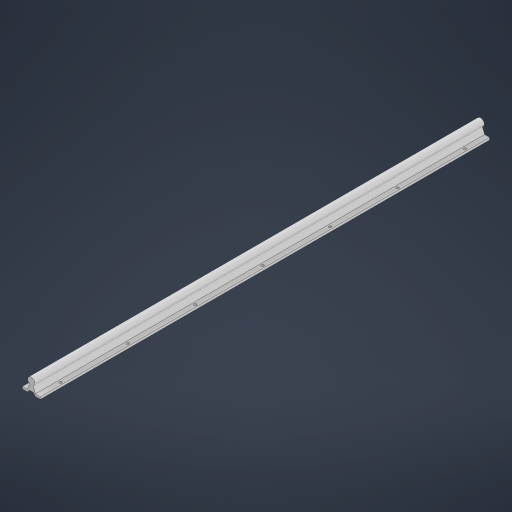
# Autodesk Inventor part: Linear Rail
Saved by Autodesk Inventor 2024 (Build 280153000, 153)
## iProperties
Created: 2024-10-26
Part Number: Linear Rail
Material: Generic
Document SubType Name: Modeling
Designer: jerem
Density: 1 g/cm^3
Appearance: Default
Author: jerem
Autodesk Inventor part; units mm, degrees
ref_plane "YZ Plane" through (0, 0, 0) normal (1, 0, 0) x (0, 1, 0)
ref_plane "XZ Plane" through (0, 0, 0) normal (0, 1, 0) x (-1, 0, 0)
ref_plane "XY Plane" through (0, 0, 0) normal (0, 0, 1) x (1, 0, 0)
sketch "Sketch1" plane through (0, 0, 0) normal (0, 0, 1) x (1, 0, 0)
  circle A0 centre (0, 0) radius 8
  line L0 (0, 0) -> (0, -24.7) construction
  line L1 (0, -24.7) -> (-19.9, -24.7)
  line L2 (-19.9, -24.7) -> (-19.9, -19.7)
  line L3 (-19.9, -19.7) -> (-9.1, -19.7)
  line L4 (-9.1, -19.7) -> (-3.85, -7.0127)
  line L5 (0, -24.7) -> (19.9, -24.7)
  line L6 (19.9, -24.7) -> (19.9, -19.7)
  line L7 (19.9, -19.7) -> (9.1, -19.7)
  line L8 (9.1, -19.7) -> (3.85, -7.0127)
  line L9 (0, 0) -> (0, 8) construction
  line L10 (-3.85, -7.0127) -> (3.85, -7.0127) construction
  line L11 (-8.85, -24.7) -> (-4.5, -19.1)
  line L12 (-4.5, -19.1) -> (0, -19.1)
  line L13 (0, -19.1) -> (4.5, -19.1)
  line L14 (4.5, -19.1) -> (8.85, -24.7)
  dimension "d0" = 16
  dimension "d1" = 39.8
  dimension "d2" = 5
  dimension "d4" = 10.8
  dimension "d7" = 32.7
  dimension "d8" = 7.7
  dimension "d9" = 9
  dimension "d10" = 5.6
  dimension "d11" = 17.7
  constraints: 30 end point, 6 equal length, 5 perpendicular, 3 horizontal, 3 point on circle, 3 point on line, 2 vertical, 1 centre point, 1 coincident
  measures "d0" diameter of A0
  measures "d1" distance between parallel lines of L6 L2
  measures "d2" distance of L1.end L2.end
  measures "d4" distance of L2.end L3.end
  measures "d7" distance of L0.end L9.end
  measures "d8" distance of L4.end L8.end
  measures "d9" distance of L13.end L11.end
  measures "d10" distance between parallel lines of L1 L12
  measures "d11" distance of L14.end L11.start
extrude "Extrusion1" add sketch "Sketch1" along normal blind 1000 contours A0 | A0 L8 L7 L6 L5 L14 L13 L12 L11 L1 L2 L3 L4
sketch "Sketch2" plane through (-19.9, -19.7, 1000) normal (0, 1, 0) x (1, 0, 0)
  circle A0 centre (5.4, 950) radius 3
  line L0 (10.8, 1000) -> (0, 1000) projected
  line L1 (5.4, 1000) -> (5.4, 950) construction
  line L2 (0, 1000) -> (11.05, 1000) construction
  point P0 (19.9, 1000)
  dimension "d14" = 50
  dimension "d15" = 6
  constraints: 2 end point, 1 centre point, 1 midpoint, 1 perpendicular
  measures "d14" distance of L1.end L1.start
  measures "d15" diameter of A0
extrude "Extrusion2" cut sketch "Sketch2" against normal through all
pattern_linear "Rectangular Pattern1" count 7 spacing 150 along (0, 0, 1) of "Extrusion2"
mirror "Mirror1" about plane through (0, 0, 0) normal (1, 0, 0) of "Rectangular Pattern1", "Extrusion2"
body "Solid1"
